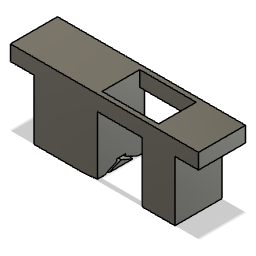
Treadmill_Chamber (Autodesk Fusion 360 design; units mm, degrees)
Autodesk Fusion 360 part; units mm, degrees
sketch "Sketch1" plane through (0, 0, 0) normal (0, 1, 0) x (1, 0, 0)
  line L0 (-25, 0) -> (15, 0)
  line L1 (15, 0) -> (15, -10)
  line L2 (15, -10) -> (-25, -10)
  line L3 (-25, -10) -> (-25, 0)
  dimension "d1" = 40
  dimension "d2" = 10
  constraint horizontal L0
  constraint vertical L1
  constraint horizontal L2
  constraint vertical L3
  measures "d1" distance of L0.start L0.end
  measures "d2" distance of L0.start L2.end
extrude "Extrude1" add sketch "Sketch1" along normal blind 16
sketch "Sketch2" plane through (0, 16, 0) normal (0, 1, 0) x (-1, 0, 0)
  line L0 (25, 10) -> (-15, 10)
  line L1 (-15, 10) -> (-15, 0)
  line L2 (-15, 0) -> (25, 0)
  line L3 (25, 0) -> (25, 10)
  line L4 (-15, 10) -> (-3, 10)
  line L5 (-3, 10) -> (-3, 9)
  line L6 (-3, 9) -> (6.5, 9)
  line L7 (6.5, 9) -> (6.5, 1)
  line L8 (6.5, 1) -> (-3, 1)
  line L9 (-3, 1) -> (-3, 9)
  dimension "d5" = 12
  dimension "d6" = 9.5
  dimension "d7" = 8
  constraint coincident L0.end L1.start
  constraint coincident L0 L4.end
  constraint perpendicular L4 L5
  constraint horizontal L6
  constraint vertical L7
  constraint horizontal L8
  constraint vertical L9
  measures "d5" distance of L0.end L4.end
  measures "d6" distance of L5.end L6.end
  measures "d7" distance of L5.end L8.end
extrude "Extrude2" cut sketch "Sketch2" against normal blind 50 contours L6 L7 L8 L9
sketch "Sketch3" plane through (0, 0, 10) normal (0, 0, 1) x (1, 0, 0)
  line L0 (-25, 0) -> (15, 0)
  line L1 (15, 0) -> (15, 16)
  line L2 (15, 16) -> (-25, 16)
  line L3 (-25, 16) -> (-25, 0)
  line L4 (15, 16) -> (3, 16)
  line L5 (3, 16) -> (3, 12.75)
  line L6 (3, 12.75) -> (-6.5, 12.75)
  line L7 (-6.5, 12.75) -> (-6.5, 16)
  line L8 (-6.5, 16) -> (3, 16)
  line L9 (3, 16) -> (3, 12.75)
  line L10 (-6.5, 12.75) -> (3, 12.75)
  line L11 (3, 12.75) -> (3, -1)
  line L12 (3, -1) -> (-6.5, -1)
  line L13 (-6.5, -1) -> (-6.5, 12.75)
  dimension "d10" = 12
  dimension "d11" = 3.25
  dimension "d12" = 9.5
  constraint coincident L1.end L2.start
  constraint coincident L2 L4.end
  constraint perpendicular L4 L5
  constraint horizontal L6
  constraint vertical L7
  constraint horizontal L8
  constraint vertical L9
  constraint coincident L2 L7.end
  constraint horizontal L10
  constraint vertical L11
  constraint horizontal L12
  constraint vertical L13
  measures "d10" distance of L1.end L4.end
  measures "d11" distance of L4.end L5.end
  measures "d12" distance of L5.end L6.end
extrude "Extrude3" cut sketch "Sketch3" against normal blind 50 contours L0 L6 L10 L11 L13
sketch "Sketch4" plane through (0, 0, 10) normal (0, 0, 1) x (1, 0, 0)
  line L0 (-6.5, 0) -> (-6.5, 12.75)
  line L1 (-6.5, 12.75) -> (3, 12.75)
  line L2 (3, 12.75) -> (3, 0)
  line L3 (3, 0) -> (15, 0)
  line L4 (15, 0) -> (15, 16)
  line L5 (15, 16) -> (-25, 16)
  line L6 (-25, 16) -> (-25, 0)
  line L7 (-25, 0) -> (-6.5, 0)
  line L8 (-25, 12.75) -> (-20, 12.75)
  line L9 (-20, 12.75) -> (-20, -3.5611)
  line L10 (-20, -3.5611) -> (-25, -3.5611)
  line L11 (-25, -3.5611) -> (-25, 12.75)
  line L12 (15, 12.75) -> (10, 12.75)
  line L13 (10, 12.75) -> (10, -3.5611)
  line L14 (10, -3.5611) -> (15, -3.5611)
  line L15 (15, -3.5611) -> (15, 12.75)
  dimension "d15" = 5
  dimension "d16" = 5
  constraint horizontal L8
  constraint vertical L9
  constraint horizontal L10
  constraint vertical L11
  constraint coincident L6 L8.start
  constraint horizontal L12
  constraint vertical L13
  constraint horizontal L14
  constraint vertical L15
  constraint coincident L4 L12.start
  measures "d15" distance of L8.start L8.end
  measures "d16" distance of L12.start L12.end
extrude "Extrude4" cut sketch "Sketch4" against normal blind 50 contours L7 L9 L10 L11 | L6 L7 L8 L9 L11 | L3 L4 L12 L13 L15 | L3 L13 L14 L15
sketch "Sketch5" plane through (0, 16, 0) normal (0, 1, 0) x (-1, 0, 0)
  line L0 (6.5, 9) -> (6.5, 1)
  line L1 (6.5, 1) -> (-3, 1)
  line L2 (-3, 1) -> (-3, 9)
  line L3 (-3, 9) -> (6.5, 9)
  line L4 (25, 10) -> (-15, 10)
  line L5 (-15, 10) -> (-15, 0)
  line L6 (-15, 0) -> (25, 0)
  line L7 (25, 0) -> (25, 10)
  line L8 (-3, 1) -> (-5.5, 1)
  line L9 (-5.5, 1) -> (-5.5, 8.9913)
  line L10 (-5.5, 8.9913) -> (-3, 8.9913)
  line L11 (-3, 8.9913) -> (-3, 1)
  dimension "d19" = 2.5
  constraint horizontal L8
  constraint vertical L9
  constraint horizontal L10
  constraint vertical L11
  constraint coincident L1.end L2.start
  measures "d19" distance of L1.end L8.end
extrude "Extrude5" cut sketch "Sketch5" against normal blind 13.5 contours L2 L8 L9 L10 L11
sketch "Sketch6" plane through (0, 0, 10) normal (0, 0, 1) x (1, 0, 0)
  line L0 (-25, 12.75) -> (-20, 12.75)
  line L1 (-20, 12.75) -> (-20, 0)
  line L2 (-20, 0) -> (-6.5, 0)
  line L3 (-6.5, 0) -> (-6.5, 12.75)
  line L4 (-6.5, 12.75) -> (3, 12.75)
  line L5 (3, 12.75) -> (3, 0)
  line L6 (3, 0) -> (10, 0)
  line L7 (10, 0) -> (10, 12.75)
  line L8 (10, 12.75) -> (15, 12.75)
  line L9 (15, 12.75) -> (15, 16)
  line L10 (15, 16) -> (-25, 16)
  line L11 (-25, 16) -> (-25, 12.75)
  line L12 (-6.5, 0) -> (-6.5, 0.3)
  line L13 (-6.5, 0) -> (-9.5, 0)
  line L14 (-9.5, 0) -> (-6.5, 0.3)
  dimension "d22" = 0.3
  dimension "d23" = 3
  constraint coincident L2.end L3.start
  constraint perpendicular L2 L12
  constraint coincident L2 L13.end
  measures "d22" distance of L2.end L12.end
  measures "d23" distance of L2.end L13.end
extrude "Extrude6" cut sketch "Sketch6" against normal blind 50 contours L2 L3 L12 L13 L14
sketch "Sketch7" plane through (3, 0, 0) normal (-1, 0, 0) x (0, 0, 1)
  line L0 (8.9913, 16) -> (8.9913, 2.5)
  line L1 (8.9913, 2.5) -> (1, 2.5)
  line L2 (1, 2.5) -> (1, 12.75)
  line L3 (1, 12.75) -> (0, 12.75)
  line L4 (0, 12.75) -> (0, 0)
  line L5 (0, 0) -> (10, 0)
  line L6 (10, 0) -> (10, 12.75)
  line L7 (10, 12.75) -> (9, 12.75)
  line L8 (9, 12.75) -> (9, 16)
  line L9 (9, 16) -> (8.9913, 16)
  line L10 (10, 0) -> (8.2, 0)
  line L11 (8.2, 0) -> (8.85, 0)
  line L12 (8.85, 0) -> (5.6472, 1.5221)
  line L13 (8.85, 0) -> (12.3961, 0) construction
  line L14 (5.6472, 1.5221) -> (4.9972, 1.5221)
  line L15 (4.9972, 1.5221) -> (8.2, 0)
  line L16 (0, 0) -> (1.8, 0)
  line L17 (1.8, 0) -> (1.15, 0)
  line L18 (1.15, 0) -> (4.3528, 1.5221)
  line L19 (4.3528, 1.5221) -> (5.0028, 1.5221)
  line L20 (4.9972, 1.5221) -> (1.8, 0)
  line L21 (4.3528, 1.5221) -> (5.6, 1.5221)
  line L22 (5.6, 1.5221) -> (5.6, 1.7721)
  line L23 (5.6, 1.7721) -> (4.3528, 1.7721)
  line L24 (4.3528, 1.7721) -> (4.3528, 1.5221)
  dimension "d26" = 1.8
  dimension "d27" = 0.65
  dimension "d28" = 154.581
  dimension "d29" = 3.5461
  dimension "d30" = 0.65
  dimension "d31" = 1.8
  dimension "d32" = 0.65
  dimension "d33" = 3.5461
  dimension "d34" = 25.419
  dimension "d35" = 0.65
  dimension "d36" = 0.25
  constraint coincident L5.end L6.start
  constraint coincident L5 L10.end
  constraint perpendicular L6 L11
  constraint horizontal L13
  constraint parallel L11 L14
  constraint coincident L4.end L5.start
  constraint coincident L5 L16.end
  constraint coincident L5 L17.end
  constraint coincident L14 L19.end
  constraint horizontal L21
  constraint vertical L22
  constraint horizontal L23
  constraint vertical L24
  measures "d26" distance of L5.end L10.end
  measures "d27" distance of L10.end L11.end
  measures "d28" angle of L12 L13
  measures "d29" distance of L11.end L12.end
  measures "d30" distance of L12.end L14.end
  measures "d31" distance of L4.end L16.end
  measures "d32" distance of L16.end L17.end
  measures "d33" distance of L17.end L18.end
  measures "d34" angle of L13 L18
  measures "d35" distance of L18.end L19.end
  measures "d36" distance of L18.end L23.end
extrude "Extrude7" cut sketch "Sketch7" along normal blind 20 and the other way blind 5 contours L5 L10 L11 L12 L14 L15 L19 L21 | L5 L16 L17 L18 L19 L20 L21 | L14 L19 L21 L22 L23 L24
sketch "Sketch8" plane through (3, 0, 0) normal (-1, 0, 0) x (0, 0, 1)
  line L0 (5.6472, 1.5221) -> (8.85, 0)
  line L1 (8.85, 0) -> (10, 0)
  line L2 (10, 0) -> (10, 12.75)
  line L3 (10, 12.75) -> (9, 12.75)
  line L4 (9, 12.75) -> (9, 16)
  line L5 (9, 16) -> (8.9913, 16)
  line L6 (8.9913, 16) -> (8.9913, 2.5)
  line L7 (8.9913, 2.5) -> (1, 2.5)
  line L8 (1, 2.5) -> (1, 12.75)
  line L9 (1, 12.75) -> (0, 12.75)
  line L10 (0, 12.75) -> (0, 0)
  line L11 (0, 0) -> (1.15, 0)
  line L12 (1.15, 0) -> (4.3528, 1.5221)
  line L13 (4.3528, 1.5221) -> (4.3528, 1.7721)
  line L14 (4.3528, 1.7721) -> (5.6, 1.7721)
  line L15 (5.6, 1.7721) -> (5.6, 1.5221)
  line L16 (5.6, 1.5221) -> (5.6472, 1.5221)
  line L17 (5.6, 1.5221) -> (8.85, 0)
  line L18 (8.85, 0) -> (8.95, 0)
  line L19 (5.6, 1.5221) -> (5.7, 1.5221)
  line L20 (5.7, 1.5221) -> (8.95, 0)
  line L21 (1.15, 0) -> (1.05, 0)
  line L22 (1.15, 0) -> (4.3528, 1.5221)
  line L23 (4.3528, 1.5221) -> (4.2528, 1.5221)
  line L24 (4.2528, 1.5221) -> (1.05, 0)
  line L25 (4.1564, 1.7721) -> (5.7264, 1.7721)
  line L26 (5.7264, 1.7721) -> (5.7264, 1.5221)
  line L27 (5.7264, 1.5221) -> (4.1564, 1.5221)
  line L28 (4.1564, 1.5221) -> (4.1564, 1.7721)
  dimension "d41" = 0.1
  dimension "d42" = 0.1
  dimension "d43" = 0.1
  dimension "d44" = 0.25
  constraint coincident L15.end L16.start
  constraint coincident L0.end L1.start
  constraint coincident L1 L18.end
  constraint perpendicular L15 L19
  constraint coincident L11.end L12.start
  constraint coincident L11 L21.end
  constraint coincident L12.end L13.start
  constraint perpendicular L13 L23
  constraint horizontal L25
  constraint vertical L26
  constraint horizontal L27
  constraint vertical L28
  measures "d41" distance of L0.end L18.end
  measures "d42" distance of L11.end L21.end
  measures "d43" distance of L12.end L23.end
  measures "d44" distance of L25.start L27.end
extrude "Extrude8" cut sketch "Sketch8" along normal blind 20 and the other way blind 5 contours L0 L16 L17 L19 L27 | L15 L16 L19 L25 L26 L27 | L13 L14 L15 L25 L27 | L13 L23 L25 L27 L28 | L11 L12 L21 L22 L23 L24 L27
sketch "Sketch9" plane through (3, 0, 0) normal (-1, 0, 0) x (0, 0, 1)
  line L0 (1.05, 0) -> (4.2528, 1.5221)
  line L1 (4.2528, 1.5221) -> (4.1564, 1.5221)
  line L2 (4.1564, 1.5221) -> (4.1564, 1.7721)
  line L3 (4.1564, 1.7721) -> (5.7264, 1.7721)
  line L4 (5.7264, 1.7721) -> (5.7264, 1.5221)
  line L5 (5.7264, 1.5221) -> (5.6472, 1.5221)
  line L6 (5.6472, 1.5221) -> (8.85, 0)
  line L7 (8.85, 0) -> (10, 0)
  line L8 (10, 0) -> (10, 12.75)
  line L9 (10, 12.75) -> (9, 12.75)
  line L10 (9, 12.75) -> (9, 16)
  line L11 (9, 16) -> (8.9913, 16)
  line L12 (8.9913, 16) -> (8.9913, 2.5)
  line L13 (8.9913, 2.5) -> (1, 2.5)
  line L14 (1, 2.5) -> (1, 12.75)
  line L15 (1, 12.75) -> (0, 12.75)
  line L16 (0, 12.75) -> (0, 0)
  line L17 (0, 0) -> (1.05, 0)
  line L18 (1.05, 0) -> (0.8, 0)
  line L19 (4.2528, 1.5221) -> (4.0028, 1.5221)
  line L20 (4.0028, 1.5221) -> (0.8, 0)
  line L21 (1.05, 0) -> (4.2528, 1.5221)
  line L22 (8.85, 0) -> (9.1, 0)
  line L23 (5.6472, 1.5221) -> (5.8972, 1.5221)
  line L24 (5.8972, 1.5221) -> (9.1, 0)
  line L25 (8.85, 0) -> (5.6472, 1.5221)
  line L26 (4.0028, 1.5221) -> (5.8972, 1.5221)
  line L27 (5.8972, 1.5221) -> (5.8972, 1.8221)
  line L28 (5.8972, 1.8221) -> (4.0028, 1.8221)
  line L29 (4.0028, 1.8221) -> (4.0028, 1.5221)
  dimension "d49" = 0.25
  dimension "d50" = 0.25
  dimension "d51" = 0.25
  dimension "d52" = 0.3
  constraint coincident L0.start L17.end
  constraint coincident L17 L18.end
  constraint parallel L17 L18
  constraint coincident L0.end L1.start
  constraint perpendicular L2 L19
  constraint coincident L6.end L7.start
  constraint perpendicular L8 L22
  constraint coincident L5.end L6.start
  constraint perpendicular L4 L23
  constraint horizontal L26
  constraint vertical L27
  constraint horizontal L28
  constraint vertical L29
  measures "d49" distance of L0.end L19.end
  measures "d50" distance of L6.end L22.end
  measures "d51" distance of L5.end L23.end
  measures "d52" distance of L19.end L28.end
extrude "Extrude9" cut sketch "Sketch9" along normal blind 20 and the other way blind 5 contours L0 L1 L17 L18 L19 L20 L21 L26 | L1 L2 L3 L4 L5 L19 L23 L26 | L2 L3 L4 L19 L23 L26 L27 L28 L29 | L5 L6 L7 L22 L23 L24 L25 L26
sketch "Sketch10" plane through (3, 0, 0) normal (-1, 0, 0) x (0, 0, 1)
  line L0 (0.8, 0) -> (4.0028, 1.5221)
  line L1 (4.0028, 1.5221) -> (4.0028, 1.8221)
  line L2 (4.0028, 1.8221) -> (5.8972, 1.8221)
  line L3 (5.8972, 1.8221) -> (5.8972, 1.5221)
  line L4 (5.8972, 1.5221) -> (9.1, 0)
  line L5 (9.1, 0) -> (10, 0)
  line L6 (10, 0) -> (10, 12.75)
  line L7 (10, 12.75) -> (9, 12.75)
  line L8 (9, 12.75) -> (9, 16)
  line L9 (9, 16) -> (8.9913, 16)
  line L10 (8.9913, 16) -> (8.9913, 2.5)
  line L11 (8.9913, 2.5) -> (1, 2.5)
  line L12 (1, 2.5) -> (1, 12.75)
  line L13 (1, 12.75) -> (0, 12.75)
  line L14 (0, 12.75) -> (0, 0)
  line L15 (0, 0) -> (0.8, 0)
  line L16 (1.8, 0) -> (5, 1.4019)
  line L17 (1.8, 0) -> (5.2936, 0) construction
  line L18 (8.2, 0) -> (5, 1.4019)
  line L19 (8.2, 0) -> (11.6936, 0) construction
  line L20 (8.2, 0) -> (8.2, 0.2)
  line L21 (8.2, 0.2) -> (4.9, 1.7)
  line L22 (4.9, 1.7) -> (1.4, 0)
  line L23 (1.4, 0) -> (1.8, 0)
  line L24 (4.0028, 1.8221) -> (4.0028, 2)
  line L25 (4.0028, 2) -> (5.9, 2)
  line L26 (5.8972, 1.8221) -> (5.9, 2)
  line L27 (5.8972, 1.8221) -> (4.0028, 1.8221)
  dimension "d57" = 23.658
  dimension "d58" = 3.4936
  dimension "d59" = 156.342
  dimension "d60" = 3.4936
  constraint horizontal L17
  constraint horizontal L19
  constraint perpendicular L19 L20
  constraint parallel L17 L23
  constraint coincident L1.end L2.start
  constraint perpendicular L2 L24
  constraint perpendicular L24 L25
  constraint coincident L2.end L3.start
  measures "d57" angle of L16 L17
  measures "d58" distance of L16.start L16.end
  measures "d59" angle of L18 L19
  measures "d60" distance of L18.start L16.end
sketch "Sketch11" plane through (3, 0, 0) normal (-1, 0, 0) x (0, 0, 1)
sketch "Sketch12" plane through (3, 0, 0) normal (-1, 0, 0) x (0, 0, 1)
  line L0 (8.2, 0) -> (4.9972, 1.5221)
  line L1 (4.9972, 1.5221) -> (1.8, 0)
  line L2 (1.8, 0) -> (8.2, 0)
  line L3 (1.8, 0) -> (4.9972, 1.5221)
  line L4 (4.9972, 1.5221) -> (8.2, 0)
  line L5 (8.2, 0) -> (5, 1.4)
  line L6 (5, 1.4) -> (1.8, 0)
  constraint coincident L1.end L2.start
  constraint coincident L0.end L1.start
  constraint coincident L0.start L2.end
extrude "Extrude10" cut sketch "Sketch10" sketch "Sketch12" along normal blind 20 and the other way blind 5 contours L2 L24 L25 L26 L27 of sketch 2 contours L0 L1 L3 L4 L5 L6
